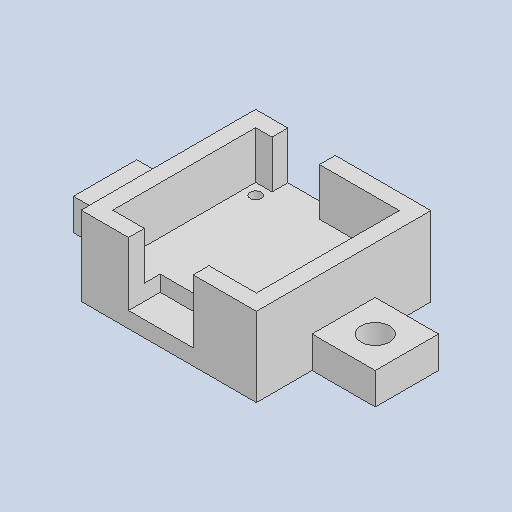
# Autodesk Inventor part: ZED-F9P-02B-case_new
Saved by Autodesk Inventor 2025.2 (Build 292293000, 293)
## iProperties
Created: 2025-05-16
Part Number: ZED-F9P-02B-case_new
Material: 일반
Document SubType Name: Modeling
Designer: jbhma
Density: 1 g/cm^3
Appearance: 기본값
Author: jbhma
Autodesk Inventor part; units mm, degrees
ref_plane "YZ Plane" through (0, 0, 0) normal (1, 0, 0) x (0, 1, 0)
ref_plane "XZ Plane" through (0, 0, 0) normal (0, 1, 0) x (-1, 0, 0)
ref_plane "XY Plane" through (0, 0, 0) normal (0, 0, 1) x (1, 0, 0)
sketch "스케치1" plane through (0, 0, 0) normal (0, 1, 0) x (-1, 0, 0)
  line L0 (27.717, -55.18) -> (-27.717, -55.18)
  line L1 (-27.717, -55.18) -> (-27.717, 0)
  line L2 (-27.717, 0) -> (27.717, 0)
  line L3 (27.717, 0) -> (27.717, -55.18)
  point P0 (0, 0)
  point P1 (0, 0)
  dimension "d0" = 55.434
  dimension "d1" = 55.18
  constraints: 8 end point, 2 parallel, 1 coincident, 1 horizontal, 1 midpoint, 1 perpendicular
  measures "d0" distance of L1.end L2.end
  measures "d1" distance of L0.end L1.end
extrude "돌출1" add sketch "스케치1" along normal blind 5
sketch "스케치2" plane through (0, 5, 0) normal (0, 1, 0) x (1, 0, 0)
  line L0 (-27.717, 0) -> (27.717, 0) projected
  line L1 (27.717, 0) -> (27.717, 55.18) projected
  line L2 (27.717, 55.18) -> (-27.717, 55.18) projected
  line L3 (-27.717, 55.18) -> (-27.717, 0) projected
  line L4 (-22.717, 50.18) -> (22.717, 50.18)
  line L5 (22.717, 50.18) -> (22.717, 5)
  line L6 (22.717, 5) -> (-22.717, 5)
  line L7 (-22.717, 5) -> (-22.717, 50.18)
  point P0 (0, 0)
  dimension "d4" = 45.434
  dimension "d5" = 45.18
  dimension "d6" = 5
  dimension "d7" = 5
  constraints: 8 end point, 2 parallel, 1 horizontal, 1 perpendicular
  measures "d4" distance of L5.end L6.end
  measures "d5" distance of L4.end L5.end
  measures "d6" distance between parallel lines of L4 L2
  measures "d7" distance between parallel lines of L3 L7
extrude "돌출2" add sketch "스케치2" along normal blind 15
sketch "스케치3" plane through (22.717, 5, -5) normal (0, 0, -1) x (-1, 0, 0)
  line L0 (45.434, 0) -> (0, 0) projected
  line L1 (45.434, 0) -> (45.434, 15) projected
  line L2 (0, 15) -> (45.434, 15) projected
  line L3 (0, 0) -> (0, 15) projected
  line L4 (15, 15) -> (35.434, 15)
  line L5 (35.434, 15) -> (35.434, 0)
  line L6 (35.434, 0) -> (15, 0)
  line L7 (15, 0) -> (15, 15)
  point P0 (22.717, -5)
  point P1 (15, 0)
  dimension "d10" = 15
  dimension "d11" = 10
  constraints: 8 end point, 2 parallel, 2 point on line, 1 horizontal, 1 perpendicular
  measures "d10" distance between parallel lines of L3 L7
  measures "d11" distance between parallel lines of L1 L5
extrude "돌출3" cut sketch "스케치3" against normal blind 15 contours L0 L7 L2 L5
sketch "스케치5" plane through (-22.717, 5, -50.18) normal (0, 0, 1) x (1, 0, 0)
  line L0 (45.434, 0) -> (0, 0) projected
  line L1 (45.434, 0) -> (45.434, 15) projected
  line L2 (0, 15) -> (45.434, 15) projected
  line L3 (0, 0) -> (0, 15) projected
  line L4 (5.2, 15) -> (20.2, 15)
  line L5 (20.2, 15) -> (20.2, 0)
  line L6 (20.2, 0) -> (5.2, 0)
  line L7 (5.2, 0) -> (5.2, 15)
  point P0 (22.717, -5)
  point P1 (5.2, 0)
  dimension "d14" = 15
  dimension "d15" = 5.2
  constraints: 8 end point, 2 parallel, 2 point on line, 1 horizontal, 1 perpendicular
  measures "d14" distance between parallel lines of L5 L7
  measures "d15" distance between parallel lines of L7 L3
extrude "돌출4" cut sketch "스케치5" against normal blind 10 contours L0 L7 L2 L5
sketch "스케치6" plane through (0, 5, 0) normal (0, 1, 0) x (1, 0, 0)
  line L0 (-22.717, 50.18) -> (-22.717, 5) projected
  line L1 (-22.717, 5) -> (-12.717, 5) projected
  line L2 (-12.717, 5) -> (-12.717, 0) projected
  line L3 (7.717, 0) -> (-12.717, 0) projected
  line L4 (7.717, 5) -> (7.717, 0) projected
  line L5 (7.717, 5) -> (22.717, 5) projected
  line L6 (22.717, 5) -> (22.717, 50.18) projected
  line L7 (22.717, 50.18) -> (-2.517, 50.18) projected
  line L8 (-2.517, 50.18) -> (-2.517, 55.18) projected
  line L9 (-17.517, 55.18) -> (-2.517, 55.18) projected
  line L10 (-17.517, 50.18) -> (-17.517, 55.18) projected
  line L11 (-17.517, 50.18) -> (-22.717, 50.18) projected
  circle A0 centre (-19.177, 46.64) radius 1.75
  circle A1 centre (19.177, 46.64) radius 1.75
  circle A2 centre (-19.177, 8.54) radius 1.75
  circle A3 centre (19.177, 8.54) radius 1.75
  point P0 (0, 0)
  dimension "d18" = 3.5
  dimension "d19" = 3.5
  dimension "d20" = 3.5
  dimension "d21" = 3.5
  dimension "d22" = 3.54
  dimension "d23" = 3.54
  dimension "d24" = 38.354
  dimension "d25" = 38.1
  dimension "d26" = 38.354
  dimension "d27" = 38.1
  dimension "d28" = 3.54
  dimension "d29" = 3.54
  dimension "d30" = 3.54
  dimension "d31" = 3.54
  dimension "d32" = 3.54
  dimension "d33" = 3.54
  constraints: 4 centre point
  measures "d18" diameter of A0
  measures "d19" diameter of A1
  measures "d20" diameter of A2
  measures "d21" diameter of A3
  measures "d22" distance from line of L11 A0.centre
  measures "d23" distance from line of A0.centre L0
  measures "d24" distance of A1.centre A0.centre
  measures "d25" distance of A2.centre A0.centre
  measures "d26" distance of A3.centre A2.centre
  measures "d27" distance of A3.centre A1.centre
  measures "d28" distance from line of L0 A2.centre
  measures "d29" distance from line of L1 A2.centre
  measures "d30" distance from line of L5 A3.centre
  measures "d31" distance from line of L6 A3.centre
  measures "d32" distance from line of L6 A1.centre
  measures "d33" distance from line of L7 A1.centre
extrude "돌출5" cut sketch "스케치6" against normal blind 10 contours A0 | A1 | A2 | A3
sketch "스케치7" plane through (27.717, 0, 0) normal (1, 0, 0) x (0, 0, -1)
  line L0 (17.59, 0) -> (37.59, 0)
  line L1 (37.59, 0) -> (37.59, 5)
  line L2 (37.59, 5) -> (17.59, 5)
  line L3 (17.59, 5) -> (17.59, 0)
  line L4 (55.18, 0) -> (55.18, 20) projected
  line L5 (0, 0) -> (0, 20) projected
  dimension "d36" = 20
  dimension "d37" = 5
  dimension "d38" = 55.18
  dimension "d39" = 17.59
  dimension "d40" = 15
  constraints: 8 end point, 2 parallel, 1 horizontal, 1 perpendicular
  measures "d36" distance of L2.end L1.end
  measures "d37" distance of L1.end L0.end
  measures "d38" distance between parallel lines of L4 L5
  measures "d39" distance between parallel lines of L3 L5
  measures "d40" distance from line of L4.end L2
extrude "돌출6" add sketch "스케치7" along normal blind 20
sketch "스케치8" plane through (27.717, 5, -17.59) normal (0, 1, 0) x (1, 0, 0)
  line L0 (0, 0) -> (0, 20) projected
  line L1 (0, 0) -> (20, 0) projected
  line L2 (20, 20) -> (20, 0) projected
  line L3 (0, 20) -> (20, 20) projected
  circle A0 centre (10, 10) radius 4.5
  point P0 (-27.717, -17.59)
  dimension "d43" = 9
  constraints: 1 centre point
  measures "d43" diameter of A0
extrude "돌출7" cut sketch "스케치8" against normal blind 20 contours A0
sketch "스케치9" plane through (-27.717, 0, -55.18) normal (-1, 0, 0) x (0, 0, 1)
  line L0 (17.59, 0) -> (37.59, 0)
  line L1 (37.59, 0) -> (37.59, 5)
  line L2 (37.59, 5) -> (17.59, 5)
  line L3 (17.59, 5) -> (17.59, 0)
  line L4 (55.18, 0) -> (55.18, 20) projected
  dimension "d46" = 20
  dimension "d47" = 5
  dimension "d48" = 17.59
  dimension "d49" = 15
  constraints: 8 end point, 2 parallel, 1 horizontal, 1 perpendicular
  measures "d46" distance of L2.end L1.end
  measures "d47" distance of L1.end L0.end
  measures "d48" distance between parallel lines of L4 L1
  measures "d49" distance from line of L4.end L2
extrude "돌출8" add sketch "스케치9" along normal blind 20
sketch "스케치10" plane through (-27.717, 5, -17.59) normal (0, 1, 0) x (1, 0, 0)
  line L0 (0, 20) -> (0, 0) projected
  line L1 (0, 20) -> (-20, 20) projected
  line L2 (-20, 0) -> (-20, 20) projected
  line L3 (0, 0) -> (-20, 0) projected
  circle A0 centre (-10, 10) radius 4.5
  point P0 (27.717, -17.59)
  dimension "d52" = 9
  constraints: 1 centre point
  measures "d52" diameter of A0
extrude "돌출9" cut sketch "스케치10" against normal blind 20 contours A0
sketch "스케치12" plane through (0, 0, 0) normal (0, -1, 0) x (1, 0, 0)
  circle A0 centre (-37.717, -27.59) radius 4.5 projected
  circle A1 centre (37.717, -27.59) radius 4.5 projected
  circle A2 centre (-19.177, -8.54) radius 1.75 projected
  circle A3 centre (19.177, -46.64) radius 1.75 projected
  circle A4 centre (19.177, -8.54) radius 1.75 projected
  circle A5 centre (-19.177, -46.64) radius 1.75 projected
  line L0 (-27.717, 0) -> (27.717, 0) projected
  line L1 (-27.717, -17.59) -> (-27.717, 0) projected
  line L2 (-27.717, -17.59) -> (-47.717, -17.59) projected
  line L3 (-47.717, -37.59) -> (-47.717, -17.59) projected
  line L4 (-27.717, -37.59) -> (-47.717, -37.59) projected
  line L5 (-27.717, -55.18) -> (-27.717, -37.59) projected
  line L6 (27.717, -55.18) -> (-27.717, -55.18) projected
  line L7 (27.717, -37.59) -> (27.717, -55.18) projected
  line L8 (27.717, -37.59) -> (47.717, -37.59) projected
  line L9 (47.717, -17.59) -> (47.717, -37.59) projected
  line L10 (27.717, -17.59) -> (47.717, -17.59) projected
  line L11 (27.717, 0) -> (27.717, -17.59) projected
  line L12 (-27.717, 0) -> (27.717, 0)
  line L13 (27.717, -55.18) -> (-27.717, -55.18)
  line L14 (27.717, -17.59) -> (47.717, -17.59)
  line L15 (47.717, -17.59) -> (47.717, -37.59)
  line L16 (47.717, -37.59) -> (27.717, -37.59)
  line L17 (-47.717, -17.59) -> (-27.717, -17.59)
  line L18 (-27.717, -37.59) -> (-47.717, -37.59)
  line L19 (-47.717, -37.59) -> (-47.717, -17.59)
  circle A6 centre (-37.717, -27.59) radius 4.5
  circle A7 centre (-19.177, -8.54) radius 1.75
  circle A8 centre (19.177, -8.54) radius 1.75
  circle A9 centre (37.717, -27.59) radius 4.5
  circle A10 centre (19.177, -46.64) radius 1.75
  circle A11 centre (-19.177, -46.64) radius 1.75
  line L20 (-27.717, -55.18) -> (-27.717, -37.59)
  line L21 (-27.717, -17.59) -> (-27.717, 0)
  line L22 (27.717, 0) -> (27.717, -17.59)
  line L23 (27.717, -37.59) -> (27.717, -55.18)
  point P0 (0, 0)
  constraints: 26 end point, 7 parallel, 6 centre point, 6 coincident, 6 concentric, 3 horizontal, 3 perpendicular
extrude "돌출10" add sketch "스케치12" along normal blind 2
sketch "스케치13" plane through (0, 5, 0) normal (0, 1, 0) x (1, 0, 0)
  circle A0 centre (-19.177, 8.54) radius 1.75 projected
  circle A1 centre (19.177, 46.64) radius 1.75 projected
  circle A2 centre (19.177, 8.54) radius 1.75 projected
  circle A3 centre (-19.177, 46.64) radius 1.75 projected
  line L0 (-22.717, 50.18) -> (-22.717, 5) projected
  line L1 (-22.717, 5) -> (-12.717, 5) projected
  line L2 (-12.717, 5) -> (-12.717, 0) projected
  line L3 (7.717, 0) -> (-12.717, 0) projected
  line L4 (7.717, 5) -> (7.717, 0) projected
  line L5 (7.717, 5) -> (22.717, 5) projected
  line L6 (22.717, 5) -> (22.717, 50.18) projected
  line L7 (22.717, 50.18) -> (-2.517, 50.18) projected
  line L8 (-2.517, 50.18) -> (-2.517, 55.18) projected
  line L9 (-17.517, 55.18) -> (-2.517, 55.18) projected
  line L10 (-17.517, 50.18) -> (-17.517, 55.18) projected
  line L11 (-17.517, 50.18) -> (-22.717, 50.18) projected
  line L12 (-12.717, 0) -> (7.717, 0)
  line L13 (7.717, 0) -> (7.717, 5)
  line L14 (-12.717, 5) -> (-12.717, 0)
  line L15 (7.717, 5) -> (7.717, 10)
  line L16 (7.717, 10) -> (-12.717, 10)
  line L17 (-12.717, 10) -> (-12.717, 5)
  point P0 (0, 0)
  dimension "d57" = 5
  constraints: 12 end point, 2 parallel, 1 horizontal, 1 perpendicular
  measures "d57" distance of L15.end L15.start
extrude "돌출11" cut sketch "스케치13" against normal blind 5 contours L17 L16 L15 L4 L3 L2
sketch "스케치14" plane through (0, -2, 0) normal (0, -1, 0) x (1, 0, 0)
  line L0 (27.717, 0) -> (-27.717, 0) projected
  line L1 (-27.717, 0) -> (-27.717, -17.59) projected
  line L2 (-27.717, -17.59) -> (-47.717, -17.59) projected
  line L3 (-47.717, -17.59) -> (-47.717, -37.59) projected
  line L4 (-47.717, -37.59) -> (-27.717, -37.59) projected
  line L5 (-27.717, -37.59) -> (-27.717, -55.18) projected
  line L6 (-27.717, -55.18) -> (27.717, -55.18) projected
  line L7 (27.717, -55.18) -> (27.717, -37.59) projected
  line L8 (27.717, -37.59) -> (47.717, -37.59) projected
  line L9 (47.717, -37.59) -> (47.717, -17.59) projected
  line L10 (47.717, -17.59) -> (27.717, -17.59) projected
  line L11 (27.717, -17.59) -> (27.717, 0) projected
  circle A0 centre (-37.717, -27.59) radius 4.5 projected
  circle A1 centre (37.717, -27.59) radius 4.5 projected
  circle A2 centre (-19.177, -8.54) radius 1.75 projected
  circle A3 centre (19.177, -46.64) radius 1.75 projected
  circle A4 centre (19.177, -8.54) radius 1.75 projected
  circle A5 centre (-19.177, -46.64) radius 1.75 projected
  line L12 (47.717, -17.59) -> (47.717, -37.59)
  line L13 (-47.717, -37.59) -> (-47.717, -17.59)
  line L14 (-27.717, 0) -> (27.717, 0)
  line L15 (27.717, -55.18) -> (-27.717, -55.18)
  circle A6 centre (-19.177, -8.54) radius 1.75
  circle A7 centre (19.177, -8.54) radius 1.75
  circle A8 centre (19.177, -46.64) radius 1.75
  circle A9 centre (-19.177, -46.64) radius 1.75
  circle A10 centre (-37.717, -27.59) radius 4.5
  circle A11 centre (37.717, -27.59) radius 4.5
  line L16 (-47.717, -17.59) -> (-27.717, -17.59)
  line L17 (27.717, -17.59) -> (47.717, -17.59)
  line L18 (47.717, -37.59) -> (27.717, -37.59)
  line L19 (-27.717, -37.59) -> (-47.717, -37.59)
  line L20 (27.717, 0) -> (27.717, -17.59)
  line L21 (27.717, -37.59) -> (27.717, -55.18)
  line L22 (-27.717, -55.18) -> (-27.717, -37.59)
  line L23 (-27.717, -17.59) -> (-27.717, 0)
  point P0 (0, 0)
  constraints: 28 end point, 10 parallel, 6 centre point, 6 coincident, 6 concentric, 4 perpendicular, 3 horizontal
extrude "돌출12" add sketch "스케치14" along normal blind 3
